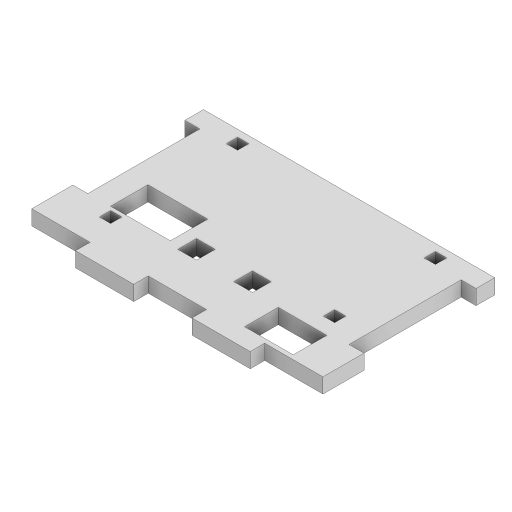
# Autodesk Inventor part: Back
Saved by Autodesk Inventor 2023.3 (Build 273359000, 359)
## iProperties
Created: 2024-06-25
Part Number: Back
Material: Generic
Document SubType Name: Modeling
Designer: David Zindović
Density: 1 g/cm^3
Appearance: Default
Author: David Zindović
Autodesk Inventor part; units mm, degrees
ref_plane "YZ Plane" through (0, 0, 0) normal (1, 0, 0) x (0, 1, 0)
ref_plane "XZ Plane" through (0, 0, 0) normal (0, 1, 0) x (-1, 0, 0)
ref_plane "XY Plane" through (0, 0, 0) normal (0, 0, 1) x (1, 0, 0)
sketch "Sketch1" plane through (0, 0, 0) normal (0, 1, 0) x (-1, 0, 0)
  line L0 (39, 19.5) -> (-39, 19.5)
  line L1 (-39, 4.6222) -> (-35, 4.6222)
  line L2 (-39, -17.5218) -> (-39, 4.6222)
  line L3 (-7.8, 19.5) -> (-23.4, 19.5)
  line L4 (-23.4, 19.5) -> (-23.4, 15.6222)
  line L5 (-23.4, 15.6222) -> (-7.8, 15.6222)
  line L6 (-7.8, 15.6222) -> (-7.8, 19.5)
  line L7 (0, 19.5) -> (0, 15.6222)
  line L8 (39, 4.6222) -> (35, 4.6222)
  line L9 (23.4, 19.5) -> (23.4, 15.6222)
  line L10 (23.4, 15.6222) -> (7.8, 15.6222)
  line L11 (7.8, 15.6222) -> (7.8, 19.5)
  line L12 (-39, 15.6222) -> (39, 15.6222)
  line L13 (39, -27.5218) -> (39, -17.5218)
  line L14 (-39, -12) -> (-39, -22)
  line L15 (-39, 4.6222) -> (-35, 4.6222)
  line L16 (-39, -27.5218) -> (-39, 4.6222)
  line L17 (35, 4.6222) -> (39, 4.6222)
  line L18 (39, 4.6222) -> (39, -25.3778)
  line L19 (-39, 19.5) -> (39, 19.5)
  line L20 (39, 19.5) -> (39, -30.3778)
  line L21 (39, -30.3778) -> (-39, -30.3778)
  line L22 (-39, -30.3778) -> (-39, 19.5)
  line L23 (-39, 4.6222) -> (-35, 4.6222)
  line L24 (-35, 4.6222) -> (-35, -25.3778)
  line L25 (-35, -25.3778) -> (-39, -25.3778)
  line L26 (-39, -25.3778) -> (-39, 4.6222)
  line L27 (35, 4.6222) -> (39, 4.6222)
  line L28 (39, 4.6222) -> (39, -25.3778)
  line L29 (39, -25.3778) -> (35, -25.3778)
  line L30 (35, -25.3778) -> (35, 4.6222)
  point P0 (0, 0)
  point P1 (39, 0)
  point P2 (-23.4, 17.5611)
  point P3 (-37, 4.6222)
  point P4 (37, 4.6222)
  point P5 (37, -27)
  point P6 (-37, -25.3778)
  point P7 (-37, 4.6222)
  dimension "d1" = 78
  dimension "d5" = 15.6
  dimension "d41" = 78
  dimension "d46" = 30
  dimension "d47" = 30
  dimension "d48" = 4
  dimension "d49" = 4
  dimension "d51" = 5
  dimension "d52" = 11
  constraints: 62 end point, 9 horizontal, 8 parallel, 7 symmetric about line, 6 midpoint, 5 perpendicular, 3 horizontal alignment, 1 point on line, 1 vertical
  measures "d1" distance of L0.start L0.end
  measures "d5" distance of L4.end L5.end
  measures "d41" distance between parallel lines of L22 L20
  measures "d46" distance of L23.end L24.end
  measures "d47" distance of L27.end L18.end
  measures "d48" distance of L24.end L25.end
  measures "d49" distance of L18.end L29.end
  measures "d51" distance between parallel lines of L21 L25
  measures "d52" distance from line of L12 point (-37, 4.622)
extrude "Extrusion1" add sketch "Sketch1" along normal mid plane 4 contours L9 L10 L11 L0 | L20 L8 L30 L29 L13 L21 L22 L16 L25 L24 L1 L12 L5 L10 | L6 L5 L4 L0
sketch "Sketch3" plane through (0, 2, 0) normal (0, 1, 0) x (1, 0, 0)
  line L0 (10, -5.5) -> (5, -5.5)
  line L1 (5, -5.5) -> (5, -0.5)
  line L2 (5, -0.5) -> (10, -0.5)
  line L3 (10, -0.5) -> (10, -5.5)
  line L4 (39, 19.5) -> (-39, 19.5) projected
  line L5 (0, 0) -> (0, -3.5827)
  line L6 (-10, -5.5) -> (-5, -5.5)
  line L7 (-5, -5.5) -> (-5, -0.5)
  line L8 (-5, -0.5) -> (-10, -0.5)
  line L9 (-10, -0.5) -> (-10, -5.5)
  line L10 (-13, -4.5) -> (-29, -4.5)
  line L11 (-29, -4.5) -> (-29, 5.5)
  line L12 (-29, 5.5) -> (-13, 5.5)
  line L13 (-13, 5.5) -> (-13, -4.5)
  line L14 (35, -8) -> (35, 22) projected
  line L15 (23.4, -15.6222) -> (39, -15.6222) projected
  line L16 (-25, -8.5) -> (-25, -5.5)
  line L17 (-25, -5.5) -> (-28, -5.5)
  line L18 (-28, -5.5) -> (-28, -8.5)
  line L19 (-28, -8.5) -> (-25, -8.5)
  line L20 (39, -15.6222) -> (39, -8) projected
  line L21 (-23.4, -19.5) -> (23.4, -19.5) projected
  line L22 (28, 25.5) -> (25, 25.5)
  line L23 (25, 25.5) -> (25, 28.5)
  line L24 (25, 28.5) -> (28, 28.5)
  line L25 (28, 28.5) -> (28, 25.5)
  line L26 (-28, 25.5) -> (-25, 25.5)
  line L27 (-25, 25.5) -> (-25, 28.5)
  line L28 (-25, 28.5) -> (-28, 28.5)
  line L29 (-28, 28.5) -> (-28, 25.5)
  line L30 (-35, 25.3778) -> (-35, -4.6222) projected
  line L31 (29.9, -14.5) -> (16.9, -14.5)
  line L32 (16.9, -14.5) -> (16.9, -5.5)
  line L33 (16.9, -5.5) -> (29.9, -5.5)
  line L34 (29.9, -5.5) -> (29.9, -14.5)
  line L35 (39, -15.6222) -> (39, -4.6222) projected
  line L36 (-39, -4.6222) -> (-39, -15.6222) projected
  line L37 (28, -1.5) -> (25, -1.5)
  line L38 (25, -1.5) -> (25, 1.5)
  line L39 (25, 1.5) -> (28, 1.5)
  line L40 (28, 1.5) -> (28, -1.5)
  point P0 (5, -3)
  point P1 (-5, -3)
  point P2 (35, 12)
  point P3 (-26.5, -8.5)
  point P4 (7.8, -19.5)
  point P5 (39, -19.5)
  point P6 (-39, -19.5)
  point P7 (35, 27)
  point P8 (26.5, 25.5)
  point P9 (-26.5, 25.5)
  point P10 (-21, -4.5)
  point P11 (23.4, -14.5)
  dimension "d9" = 5
  dimension "d10" = 5
  dimension "d11" = 5
  dimension "d12" = 20
  dimension "d13" = 16
  dimension "d14" = 10
  dimension "d53" = 3
  dimension "d54" = 3
  dimension "d56" = 6
  dimension "d57" = 15
  dimension "d58" = 13
  dimension "d59" = 9
  dimension "d61" = 5
  dimension "d62" = 3
  dimension "d63" = 3
  dimension "d64" = 11
  dimension "d65" = 11
  dimension "d66" = 3
  dimension "d67" = 3
  dimension "d68" = 11
  dimension "d69" = 18
  constraints: 66 end point, 10 symmetric about line, 9 parallel, 5 horizontal, 5 perpendicular, 4 midpoint, 1 vertical, 1 vertical alignment
  measures "d9" distance of L1.end L2.end
  measures "d10" distance of L0.end L1.end
  measures "d11" horizontal distance of L5.start point (5, -3)
  measures "d12" distance between parallel lines of L4 L2
  measures "d13" distance of L11.end L12.end
  measures "d14" distance of L10.end L11.end
  measures "d53" distance of L23.end L24.end
  measures "d54" distance of L22.end L23.end
  measures "d56" distance between parallel lines of L30 L11
  measures "d57" distance from line of L21 point (-21, -4.5)
  measures "d58" distance of L32.end L33.end
  measures "d59" distance of L31.end L32.end
  measures "d61" distance between parallel lines of L21 L31
  measures "d62" distance of L18.end L16.start
  measures "d63" distance of L17.end L18.end
  measures "d64" distance between parallel lines of L36 L18
  measures "d65" distance between parallel lines of L21 L19
  measures "d66" distance of L38.end L39.end
  measures "d67" distance of L37.end L38.end
  measures "d68" distance between parallel lines of L20 L40
  measures "d69" distance between parallel lines of L21 L37
extrude "Extrusion2" cut sketch "Sketch3" against normal up to surface (4 mm away)
sketch "Sketch4" plane through (0, 2, 0) normal (0, 1, 0) x (1, 0, 0)
  line L0 (39, 34.5) -> (-39, 34.5) projected
  line L1 (-39, 30.3778) -> (-39, 22) projected
  line L2 (39, 34.5) -> (-39, 34.5)
  line L3 (-39, 34.5) -> (-39, 30.5)
  line L4 (-39, 30.5) -> (39, 30.5)
  line L5 (39, 30.5) -> (39, 34.5)
  point P0 (0, 0)
  point P1 (-39, 27)
  dimension "d29" = 4
  constraints: 8 end point, 2 parallel, 1 horizontal, 1 perpendicular, 1 point on line
  measures "d29" distance of L3.end L2.end
extrude "Extrusion3" [suppressed]
equation "\"d5\" = 0.2 * d1"
equation "\"d9\" = d10"
body "Solid1"
